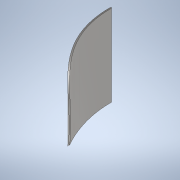
# Autodesk Inventor part: труба
Saved by Autodesk Inventor 2020.1 (Build 241239000, 239)
## iProperties
Created: 2021-07-14
Part Number: труба
Material: Нержавеющая сталь
Document SubType Name: ЛистМат
Designer: Ni3na
Density: 8 g/cm^3
Appearance: С умеренной полировкой
Sheet Metal Rule: По умолчанию
Flat Pattern Width: 14.6521 cm
Flat Pattern Length: 12.5 cm
Flat Pattern Area: 183.151 cm^2
Sheet Metal Width: 146,521 мм
Sheet Metal Length: 125,000 мм
Sheet Metal Area: 18315,147 мм^2
Author: Ni3na
Autodesk Inventor part; units mm, degrees
ref_plane "YZ Plane" through (0, 0, 0) normal (1, 0, 0) x (0, 1, 0)
ref_plane "XZ Plane" through (0, 0, 0) normal (0, 1, 0) x (-1, 0, 0)
ref_plane "XY Plane" through (0, 0, 0) normal (0, 0, 1) x (1, 0, 0)
sketch "Эскиз1" plane through (0, 0, 0) normal (0, 0, 1) x (1, 0, 0)
  line L0 (0, 0) -> (125, 0)
  line L1 (125, 0) -> (125, -125)
  line L2 (125, -125) -> (0, -125)
  line L3 (0, -125) -> (0, 0)
  dimension "d0" = 125
  dimension "d1" = 125
  constraints: 8 end point, 2 parallel, 1 horizontal, 1 perpendicular
  measures "d0" distance of L0.start L0.end
  measures "d1" distance of L2.end L0.start
extrude "Выдавливание1" add sketch "Эскиз1" along normal blind 300
sketch "Эскиз2" plane through (125, -125, 0) normal (1, 0, 0) x (0, 0, -1)
  line L0 (0, 0) -> (-300, 0) projected
  line L1 (0, 125) -> (-300, 125) projected
  line L2 (-212.5, 0) -> (-87.5, 0)
  line L3 (-87.5, 0) -> (-87.5, 125)
  line L4 (-87.5, 125) -> (-212.5, 125)
  line L5 (-212.5, 125) -> (-212.5, 0)
  point P0 (-150, 0)
  point P1 (-150, 0)
  point P2 (-212.5, 125)
  point P3 (-87.5, 0)
  dimension "d4" = 125
  dimension "d5" = 0
  constraints: 8 end point, 2 midpoint, 2 parallel, 2 point on line, 1 horizontal, 1 perpendicular
  measures "d4" distance of L4.end L3.end
  measures "d5" distance of point (-150, 0) point (-150, 0)
extrude "Выдавливание2" add sketch "Эскиз2" along normal blind 82.5
sketch "Эскиз9" plane through (0, 0, 0) normal (0, 1, 0) x (1, 0, 0)
  line L0 (125, -212.5) -> (125, -300) projected
  line L1 (125, -279.9507) -> (0, -279.9507)
  line L2 (0, 0) -> (0, -300) projected
  line L3 (125, -87.5) -> (207.5, -87.5) projected
  line L4 (125, -87.5) -> (0, -87.5)
  circle A0 centre (218.75, -87.5) radius 156.25
  circle A1 centre (218.75, -87.5) radius 155.25
  circle A2 centre (218.75, -87.5) radius 157.25
  line L5 (125, -212.5) -> (207.5, -212.5) projected
  line L6 (125, -212.5) -> (207.5, -212.5)
  line L7 (207.5, -212.5) -> (125, -212.5)
  line L8 (125, -212.5) -> (125, -224.7107)
  line L9 (0, -279.9507) -> (125, -279.9507)
  line L10 (125, -279.9507) -> (125, -300)
  line L11 (125, -300) -> (0, -300)
  line L12 (0, -300) -> (0, -279.9507)
  circle A3 centre (62.5, -87.5) radius 1
  point P0 (63.5, -87.5)
  point P1 (61.5, -87.5)
  point P2 (125, -213.7478)
  point P3 (126.6763, -212.5)
  point P4 (63.5, -87.5)
  dimension "d19" = 93.75
  dimension "d20" = 1
  dimension "d21" = 1
  constraints: 18 end point, 6 point on line, 5 coincident, 4 equal length, 2 horizontal, 2 perpendicular, 1 horizontal alignment, 1 midpoint, 11 other
  measures "d19" distance of point (218.75, -87.5) L3.start
  measures "d20" distance of point (63.5, -87.5) point (62.5, -87.5)
  measures "d21" distance of point (62.5, -87.5) point (61.5, -87.5)
extrude "Выдавливание6" cut sketch "Эскиз9" against normal blind 200 contours L0 L11 L2 L1 | A2 A3 A0 L0 | A0 A3 A1 L5 | A3 A0 L4 | L4 A0 A3 | A0 L4 A3 | A0 A3 L4 keep common part picked at (62.7561, -98.9034) picked at (121.9581, -209.089)
sketch "Эскиз11" plane through (0, 0, 300) normal (0, 0, 1) x (1, 0, 0)
  line L0 (125, 0) -> (0, 0) projected
  line L1 (0, -125) -> (0, 0) projected
  circle A0 centre (62.5, -62.5) radius 62.5
  point P0 (62.5, 0)
  point P1 (0, -62.5)
  constraints: 2 midpoint, 1 vertical alignment, 2 other
extrude "Выдавливание7" cut sketch "Эскиз11" against normal blind 300 contours A0 keep common part
sketch "Эскиз12" plane through (62.5, -62.5, 300) normal (0, 0, 1) x (1, 0, 0)
  circle A0 centre (-10.575, 6.8149) radius 127.9609
  point P0 (-62.5, 62.5)
  constraints: 1 centre point
extrude "Выдавливание8" cut sketch "Эскиз12" against normal blind 30
equation "\"Радиус_гибки\" = Толщина"
equation "\"Ширина_просечки\" = Толщина"
equation "\"Глубина_просечки\" = 0.5 * Толщина"
equation "\"Размер_просечки\" = 4 * Толщина"
equation "\"Мин_остаток\" = 2 * Толщина"
equation "\"Радиус_перехода\" = Радиус_гибки"
equation "\"Радиус_Якоби\" = Толщина"
equation "\"Размер_зазора\" = Толщина"
equation "\"Толщина\" = 2"
